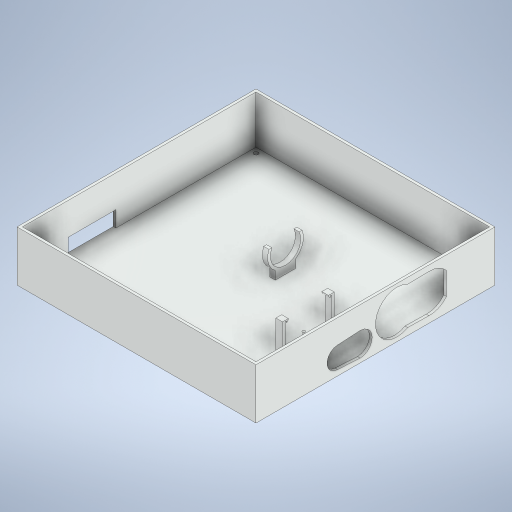
# Autodesk Inventor part: base plate
Saved by Autodesk Inventor 2024.1 (Build 281209000, 209)
## iProperties
Created: 2025-03-25
Part Number: base plate
Material: Generic
Document SubType Name: Modeling
Designer: User
Density: 1 g/cm^3
Appearance: Default
Author: User
Autodesk Inventor part; units mm, degrees
ref_plane "YZ Plane" through (0, 0, 0) normal (1, 0, 0) x (0, 1, 0)
ref_plane "XZ Plane" through (0, 0, 0) normal (0, 1, 0) x (-1, 0, 0)
sketch "Sketch1" plane through (0, 0, 0) normal (0, 1, 0) x (-1, 0, 0)
  line L0 (0, 0) -> (180, 0)
  line L1 (180, 0) -> (180, -180)
  line L2 (180, -180) -> (0, -180)
  line L3 (0, -180) -> (0, 0)
  dimension "d0" = 180
  dimension "d1" = 180
  constraints: 8 end point, 2 parallel, 1 horizontal, 1 perpendicular
  measures "d0" distance of L1.end L2.end
  measures "d1" distance of L0.end L1.end
extrude "Extrusion1" add sketch "Sketch1" along normal blind 2
sketch "Sketch4" plane through (0, 2, 0) normal (0, 1, 0) x (1, 0, 0)
  line L0 (0, 180) -> (-180, 180) projected
  line L1 (-180, 180) -> (-180, 0) projected
  line L2 (0, 180) -> (-180, 180)
  line L3 (-180, 180) -> (-180, 178)
  line L4 (-180, 178) -> (0, 178)
  line L5 (0, 178) -> (0, 180)
  line L6 (-180, 0) -> (0, 0) projected
  line L7 (0, 0) -> (-180, 0)
  line L8 (-180, 0) -> (-180, 2)
  line L9 (-180, 2) -> (0, 2)
  line L10 (0, 2) -> (0, 0)
  line L11 (0, 2) -> (-2, 2)
  line L12 (-2, 2) -> (-2, 178)
  line L13 (-2, 178) -> (0, 178)
  line L14 (0, 178) -> (0, 2)
  line L15 (-180, 178) -> (-178, 178)
  line L16 (-178, 178) -> (-178, 2)
  line L17 (-178, 2) -> (-180, 2)
  line L18 (-180, 2) -> (-180, 178)
  dimension "d16" = 2
  dimension "d17" = 2
  dimension "d18" = 2
  dimension "d19" = 2
  constraints: 32 end point, 8 parallel, 4 horizontal, 4 perpendicular, 4 point on line
  measures "d16" distance of L3.end L2.end
  measures "d17" distance of L7.end L8.end
  measures "d18" distance of L12.end L13.end
  measures "d19" distance of L16.end L17.end
extrude "Extrusion4" add sketch "Sketch4" along normal blind 36 contours L5 L4 L1 L0 | L14 L9 L12 L4 | L4 L16 L9 L1 | L10 L6 L1 L9
sketch "Sketch5" plane through (0, 2, 0) normal (0, 1, 0) x (1, 0, 0)
  circle A0 centre (-174, 6) radius 1.65
  circle A1 centre (-174, 174) radius 1.65
  circle A2 centre (-6, 174) radius 1.65
  circle A3 centre (-6, 6) radius 1.65
  point P0 (0, 0)
  dimension "d22" = 3.3
  dimension "d23" = 3.3
  dimension "d24" = 3.3
  dimension "d25" = 3.3
  constraints: 4 centre point
  measures "d22" diameter of A0
  measures "d23" diameter of A1
  measures "d24" diameter of A2
  measures "d25" diameter of A3
extrude "Extrusion5" cut sketch "Sketch5" against normal through all
sketch "Sketch8" plane through (-180, 0, -180) normal (-1, 0, 0) x (0, 0, 1)
  line L0 (178, 2) -> (2, 2) projected
  line L1 (143.5, 14) -> (107.5, 14)
  line L2 (107.5, 14) -> (107.5, 2)
  line L3 (107.5, 2) -> (143.5, 2)
  line L4 (143.5, 2) -> (143.5, 14)
  line L5 (178, 2) -> (178, 38) projected
  point P0 (180, 0)
  point P1 (143.5, 2)
  point P2 (107.5, 2)
  dimension "d84" = 36
  dimension "d101" = 12
  dimension "d108" = 34.5
  constraints: 8 end point, 2 parallel, 1 horizontal, 1 perpendicular
  measures "d84" distance of L3.end L2.end
  measures "d101" distance of L1.end L2.end
  measures "d108" distance between parallel lines of L5 L4
extrude "Extrusion10" cut sketch "Sketch8" against normal blind 10
sketch "Sketch15" plane through (-2, 2, -2) normal (-1, 0, 0) x (0, 0, 1)
  line L0 (-141.5, 17.33) -> (-133.04, 17.33) construction
  line L1 (-112.2541, 3.188) -> (-128.2862, 2.9082)
  arc A0 (-141.5, 8.8698) -> (-128.2862, 2.9082) centre (-129.027, 18.891) ccw
  arc A1 (-112.2541, 3.188) -> (-88, 17.33) centre (-104.25, 17.33) ccw
  line L2 (-112.2541, 31.472) -> (-128.2862, 31.7518)
  arc A2 (-128.2862, 31.7518) -> (-141.5, 25.7902) centre (-129.027, 15.769) ccw
  arc A3 (-88, 17.33) -> (-112.2541, 31.472) centre (-104.25, 17.33) ccw
  line L3 (-141.5, 17.33) -> (-141.5, 8.8698)
  line L4 (-141.5, 17.33) -> (-141.5, 25.7902)
  line L5 (-176, 36) -> (0, 36) projected
  line L6 (0, 0) -> (-176, 0) projected
  point P0 (2, -2)
  constraints: 10 end point, 8 point on circle, 4 centre point, 1 horizontal, 1 vertical
extrude "Extrusion17" cut sketch "Sketch15" against normal through all
ref_plane "Work Plane1" through (-84, 2, -178) normal (-1, 0, 0) x (0, 0, 1)
sketch "Sketch16" plane through (-84, 2, -178) normal (-1, 0, 0) x (0, 0, 1)
  arc A0 (63.7459, 3.188) -> (63.7459, 31.472) centre (71.75, 17.33) ccw projected
  line L0 (176, 0) -> (0, 0) projected
  line L1 (71.75, 0) -> (79.5, 0)
  line L2 (-2, -2) -> (178, -2) projected
  line L3 (45.25, 0) -> (53, 0) construction
  line L4 (79.5, 0) -> (79.5, 6.2762)
  line L5 (71.75, 0) -> (64, 0)
  line L6 (45.25, 0) -> (53, 0) construction
  line L7 (64, 0) -> (64, 6.2762)
  arc A1 (61.4422, 22.429) -> (82.0578, 22.429) centre (71.75, 17.33) ccw
  line L8 (59.25, 22.429) -> (61.4422, 22.429)
  line L9 (82.0578, 22.429) -> (84.25, 22.429)
  arc A2 (59.25, 22.429) -> (64, 6.2762) centre (71.75, 17.33) ccw
  arc A3 (79.5, 6.2762) -> (84.25, 22.429) centre (71.75, 17.33) ccw
  dimension "d135" = 23
  constraints: 16 end point, 6 point on circle, 3 centre point, 3 collinear, 2 horizontal, 2 point on line, 1 coincident, 1 parallel
  measures "d135" diameter of A1
extrude "Extrusion18" add sketch "Sketch16" along normal blind 4
sketch "Sketch17" plane through (0, 0, 0) normal (1, 0, 0) x (0, 0, -1)
  line L0 (36.5, 2) -> (2, 2) projected
  line L1 (53, 2) -> (88, 2)
  line L2 (88, 2) -> (88, 23.37)
  line L3 (88, 23.37) -> (53, 23.37)
  line L4 (53, 23.37) -> (53, 2)
  line L5 (0, 0) -> (0, 38) projected
  arc A0 (61.49, 20.185) -> (61.49, 4.185) centre (61.49, 12.185) ccw
  arc A1 (77.4348, 3.2471) -> (77.4348, 21.1229) centre (78.49, 12.185) ccw
  line L6 (78.49, 3.185) -> (61.49, 4.185)
  line L7 (78.49, 21.185) -> (61.49, 20.185)
  dimension "d144" = 35
  dimension "d145" = 21.37
  dimension "d147" = 16
  dimension "d148" = 18
  constraints: 12 end point, 6 point on circle, 2 centre point, 2 parallel, 2 point on line, 1 horizontal, 1 perpendicular
  measures "d144" distance of L3.end L2.end
  measures "d145" distance of L2.end L1.end
  measures "d147" diameter of A0
  measures "d148" diameter of A1
extrude "Extrusion19" cut sketch "Sketch17" against normal blind 10 contours L7 A1 L6 A0
sketch "Sketch21" plane through (0, 2, 0) normal (0, 1, 0) x (1, 0, 0)
  circle A0 centre (-17.39, 69.81) radius 1.05
  circle A1 centre (-33.79, 69.81) radius 1.05
  point P0 (0, 0)
  dimension "d155" = 2.1
  dimension "d156" = 2.1
  constraints: 2 centre point
  measures "d155" diameter of A0
  measures "d156" diameter of A1
extrude "Extrusion21" add sketch "Sketch21" along normal blind 6
sketch "Sketch22" plane through (0, 2, 0) normal (0, 1, 0) x (1, 0, 0)
  line L0 (-36, 88) -> (-31, 88)
  line L1 (-31, 88) -> (-31, 90)
  line L2 (-31, 90) -> (-36, 90)
  line L3 (-36, 90) -> (-36, 88)
  line L4 (-31, 53) -> (-36, 53)
  line L5 (-36, 53) -> (-36, 51)
  line L6 (-36, 51) -> (-31, 51)
  line L7 (-31, 51) -> (-31, 53)
  line L8 (-2, 2) -> (-2, 178) projected
  line L9 (-2, 90) -> (-178, 90) construction
  line L10 (-178, 178) -> (-178, 72.5) projected
  point P0 (0, 0)
  dimension "d159" = 5
  dimension "d160" = 2
  dimension "d161" = 5
  dimension "d162" = 2
  constraints: 18 end point, 4 parallel, 3 horizontal, 2 perpendicular, 2 point on line, 1 midpoint
  measures "d159" distance of L2.end L1.end
  measures "d160" distance of L1.end L0.end
  measures "d161" distance of L6.end L5.end
  measures "d162" distance of L5.end L4.end
extrude "Extrusion22" add sketch "Sketch22" along normal blind 23
sketch "Sketch23" plane through (-36, 2, -88) normal (0, 0, 1) x (1, 0, 0)
  line L0 (5, 0) -> (5, 23) projected
  line L1 (5, 23) -> (0, 23)
  line L2 (0, 23) -> (0, 21)
  line L3 (0, 21) -> (5, 21)
  line L4 (5, 21) -> (5, 23)
  point P0 (36, -2)
  dimension "d165" = 5
  dimension "d166" = 2
  constraints: 8 end point, 2 parallel, 1 horizontal, 1 perpendicular
  measures "d165" distance of L3.end L2.end
  measures "d166" distance of L2.end L1.end
sketch "Sketch24" plane through (-31, 2, -53) normal (0, 0, -1) x (-1, 0, 0)
  line L0 (0, 23) -> (5, 23)
  line L1 (5, 23) -> (5, 21)
  line L2 (5, 21) -> (0, 21)
  line L3 (0, 21) -> (0, 23)
  point P0 (-31, -2)
  dimension "d167" = 5
  dimension "d168" = 2
  constraints: 8 end point, 2 parallel, 1 horizontal, 1 perpendicular
  measures "d167" distance of L1.end L2.end
  measures "d168" distance of L0.end L1.end
extrude "Extrusion23" add sketch "Sketch23" along normal blind 2.4
extrude "Extrusion24" add sketch "Sketch24" along normal blind 2.4
sketch "Sketch25" plane through (-36, 23, -88) normal (0, -1, 0) x (1, 0, 0)
  line L0 (5, 0) -> (0, 0)
  line L1 (0, 0) -> (0, 1.2)
  line L2 (0, 1.2) -> (5, 1.2)
  line L3 (5, 1.2) -> (5, 0)
  point P0 (36, 88)
  dimension "d173" = 5
  dimension "d174" = 1.2
  constraints: 8 end point, 2 parallel, 1 horizontal, 1 perpendicular
  measures "d173" distance of L1.end L2.end
  measures "d174" distance of L0.end L1.end
sketch "Sketch26" plane through (-36, 23, -53) normal (0, -1, 0) x (1, 0, 0)
  line L0 (5, 0) -> (0, 0)
  line L1 (0, 0) -> (0, -1.2)
  line L2 (0, -1.2) -> (5, -1.2)
  line L3 (5, -1.2) -> (5, 0)
  point P0 (36, 53)
  dimension "d175" = 5
  dimension "d176" = 1.2
  constraints: 8 end point, 2 parallel, 1 horizontal, 1 perpendicular
  measures "d175" distance of L2.end L1.end
  measures "d176" distance of L1.end L0.end
extrude "Extrusion25" cut sketch "Sketch26" against normal blind 1
extrude "Extrusion26" cut sketch "Sketch25" against normal blind 1
fillet "Fillet1" radius 2.5 2 edges at (-33.5, 23, -85.6) (-33.5, 23, -55.4)
body "Solid1"
